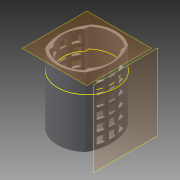
# Autodesk Inventor part: Lattice
Saved by Autodesk Inventor 2013 (Build 170138000, 138)
## iProperties
Created: 2014-07-04
Part Number: Lattice
Material: Genérico
Document SubType Name: Chapa
Designer: Administrador
Density: 1 g/cm^3
Sheet Metal Rule: Por defecto_mm
Author: Administrador
Autodesk Inventor part; units mm, degrees
ref_plane "XZ Plane" through (0, 0, 0) normal (0, 1, 0) x (-1, 0, 0)
ref_plane "XY Plane" through (0, 0, 0) normal (0, 0, 1) x (1, 0, 0)
sketch "Boceto1" plane through (0, 0, 0) normal (0, 0, 1) x (1, 0, 0)
  circle A0 centre (0, 0) radius 20.1
  circle A1 centre (0, 0) radius 18.1
  line L0 (-13, 22.4256) -> (13, 22.4256)
  line L1 (13, 22.4256) -> (13, -22.4256)
  line L2 (13, -22.4256) -> (-13, -22.4256)
  line L3 (-13, -22.4256) -> (-13, 22.4256)
  line L4 (-13, 22.4256) -> (13, -22.4256) construction
  line L5 (13, 22.4256) -> (-13, -22.4256) construction
  circle A2 centre (0, 0) radius 22.1
  dimension "d0" = 40.2
  dimension "d1" = 36.2
  dimension "d2" = 26
  dimension "d3" = 44.2
  constraints: 12 end point, 3 centre point, 2 midpoint, 2 parallel, 1 horizontal, 1 perpendicular
  measures "d0" diameter of A0
  measures "d1" diameter of A1
  measures "d2" distance of L1.end L2.end
  measures "d3" diameter of A2
extrude "Extrusión1" add sketch "Boceto1" along normal blind 10 contours A0 L1 A1 | A0 L1 A2 | L1 A1 L3 A0 | A0 L3 A2 L1 | L1 A2 L3 A0 | A0 L3 A1 L1 | L3 A1 A0 | A0 L3 A2
sketch "Boceto2" plane through (0, 0, 10) normal (0, 0, 1) x (1, 0, 0)
  line L0 (-13.4694, 30.192) -> (13.3129, 30.192)
  line L1 (13.3129, 30.192) -> (13.3129, -30.5468)
  line L2 (13.3129, -30.5468) -> (-13.4694, -30.5468)
  line L3 (-13.4694, -30.5468) -> (-13.4694, 30.192)
  line L4 (-13.4694, 30.192) -> (13.3129, -30.5468) construction
  line L5 (13.3129, 30.192) -> (-13.4694, -30.5468) construction
  circle A0 centre (0, 0) radius 22.0966
  line L6 (-13, 18.1) -> (-15.3267, 9.6283)
  line L7 (13, 18.1) -> (15.412, 9.491)
  line L8 (13, -18.1) -> (15.608, -9.1652)
  line L9 (-13, -18.1) -> (-15.3267, -9.1652)
  arc A1 (13.3129, 15.0591) -> (-13.4694, 14.9193) centre (0, 0) ccw
  arc A2 (14.1027, -14.3221) -> (14.0417, 14.382) centre (0, 0) ccw
  arc A3 (-14.0136, 14.4093) -> (-13.9434, -14.4773) centre (0, 0) ccw
  arc A4 (-13.4694, -14.9193) -> (13.3129, -15.0591) centre (0, 0) ccw
  point P0 (-0.0782, -0.1774)
  dimension "d32" = 26.7823
  constraints: 20 end point, 8 point on circle, 8 point on line, 5 centre point, 2 midpoint, 2 parallel, 1 horizontal, 1 perpendicular
  measures "d32" distance of L1.end L2.end
extrude "Extrusión2" cut sketch "Boceto2" against normal through all contours A1 L1 A4 L3
sketch "Boceto3" plane through (0, 0, 10) normal (0, 0, 1) x (1, 0, 0)
  circle A0 centre (0, 0) radius 22.1 projected
  line L0 (13.3129, -12.2628) -> (13.3129, -15.0591) projected
  arc A1 (-13.4694, -14.9193) -> (13.3129, -15.0591) centre (0, 0) ccw projected
  line L1 (-13.4694, -14.9193) -> (-13.4694, -12.0907) projected
  arc A2 (-13.4694, 12.0907) -> (-13.4694, -12.0907) centre (0, 0) ccw projected
  line L2 (-13.4694, 12.0907) -> (-13.4694, 14.9193) projected
  arc A3 (13.3129, 15.0591) -> (-13.4694, 14.9193) centre (0, 0) ccw projected
  line L3 (13.3129, 15.0591) -> (13.3129, 12.2628) projected
  arc A4 (13.3129, -12.2628) -> (13.3129, 12.2628) centre (0, 0) ccw projected
ref_plane "Plano de trabajo1" through (0, 0, 24.5) normal (0, 0, 1) x (1, 0, 0)
sketch "Boceto5" plane through (0, 0, 24.5) normal (0, 0, 1) x (1, 0, 0)
  circle A0 centre (0, 0) radius 22.1 projected
  arc A1 (13.3129, 15.0591) -> (-13.4694, 14.9193) centre (0, 0) ccw projected
  line L0 (-13.4694, 12.0907) -> (-13.4694, 14.9193) projected
  arc A2 (-13.4694, 12.0907) -> (-13.4694, -12.0907) centre (0, 0) ccw projected
  line L1 (-13.4694, -14.9193) -> (-13.4694, -12.0907) projected
  arc A3 (-13.4694, -14.9193) -> (13.3129, -15.0591) centre (0, 0) ccw projected
  line L2 (13.3129, -12.2628) -> (13.3129, -15.0591) projected
  arc A4 (13.3129, -12.2628) -> (13.3129, 12.2628) centre (0, 0) ccw projected
  line L3 (13.3129, 15.0591) -> (13.3129, 12.2628) projected
  line L4 (-0.172, 27.8672) -> (-0.172, -32.3033)
  arc A5 (13.2871, -19.3756) -> (13.9152, 16.5315) centre (0.9992, -1.2016) ccw
  arc A6 (-12.5238, 19.0209) -> (-13.9692, -18.7386) centre (12.6013, -0.8483) ccw
  arc A7 (-12.5238, 19.0209) -> (-13.9692, -18.7386) centre (-2.0748, -0.2865) ccw
  arc A8 (13.6252, -18.7386) -> (12.1797, 19.0209) centre (-12.9453, -0.8483) ccw
  arc A9 (13.6252, -18.7386) -> (12.1797, 19.0209) centre (1.7308, -0.2865) ccw
  constraints: 10 point on circle, 5 centre point, 4 symmetric about line, 2 end point, 2 other
extrude "Extrusión4" cut sketch "Boceto5" against normal through all contours A0 A8 A5 | A0 A5 A9 A8 | A5 A8 A0 | A0 A8 A9 A5 | A6 A7 A0 | A0 A6
sketch "Boceto6" plane through (0, 0, 24.5) normal (0, 0, 1) x (1, 0, 0)
  line L0 (13.3129, -12.2628) -> (13.3129, -15.0591) projected
  arc A0 (-13.4694, -14.9193) -> (13.3129, -15.0591) centre (0, 0) ccw projected
  line L1 (-13.4694, -14.9193) -> (-13.4694, -12.0907) projected
  arc A1 (-13.4694, 12.0907) -> (-13.4694, -12.0907) centre (0, 0) ccw projected
  line L2 (-13.4694, 12.0907) -> (-13.4694, 14.9193) projected
  arc A2 (13.3129, 15.0591) -> (-13.4694, 14.9193) centre (0, 0) ccw projected
  line L3 (13.3129, 15.0591) -> (13.3129, 12.2628) projected
  arc A3 (13.3129, -12.2628) -> (13.3129, 12.2628) centre (0, 0) ccw projected
  arc A4 (15.3099, -15.9379) -> (13.0991, 17.7996) centre (-12.9453, -0.8483) ccw projected
  arc A5 (13.0991, 17.7996) -> (-13.844, 17.2266) centre (0, 0) ccw projected
  arc A6 (-13.844, 17.2266) -> (-16.028, -15.2156) centre (12.6013, -0.8483) ccw projected
  arc A7 (-16.028, -15.2156) -> (15.3099, -15.9379) centre (0, 0) ccw projected
extrude "Extrusión5" add sketch "Boceto6" against normal blind 52
ref_plane "Plano de trabajo2" through (29, 0, 0) normal (1, 0, 0) x (0, 1, 0)
sketch "Boceto7" plane through (29, 0, 0) normal (1, 0, 0) x (0, 1, 0)
  line L0 (17.7996, 24.5) -> (-15.9379, 24.5) projected
  line L1 (-15.2156, 24.5) -> (-22.1, 24.5) projected
  line L2 (-22.1, -27.5) -> (-22.1, 24.5) projected
  line L3 (22.1, -27.5) -> (22.1, 24.5) projected
  line L4 (22.1, 24.5) -> (17.2266, 24.5) projected
  line L5 (-15.9379, -27.5) -> (17.7996, -27.5) projected
  line L6 (17.2266, -27.5) -> (22.1, -27.5) projected
  line L7 (-22.1, -27.5) -> (-15.2156, -27.5) projected
  line L8 (-15.9379, -27.5) -> (-15.9379, 24.5) projected
  line L9 (17.7996, 24.5) -> (17.7996, -27.5) projected
  line L10 (-12.0907, 24.5) -> (-12.0907, -27.5) projected
  line L11 (12.0907, -27.5) -> (12.0907, 24.5) projected
  line L12 (-10.3756, 20.6878) -> (-5.3756, 20.6878)
  line L13 (-5.3756, 20.6878) -> (-5.3756, 15.6878)
  line L14 (-5.3756, 15.6878) -> (-10.3756, 15.6878)
  line L15 (-10.3756, 15.6878) -> (-10.3756, 20.6878)
  line L16 (-2.3756, 20.6878) -> (2.6244, 20.6878)
  line L17 (2.6244, 20.6878) -> (2.6244, 15.6878)
  line L18 (2.6244, 15.6878) -> (-2.3756, 15.6878)
  line L19 (-2.3756, 15.6878) -> (-2.3756, 20.6878)
  line L20 (5.6244, 20.6878) -> (10.6244, 20.6878)
  line L21 (10.6244, 20.6878) -> (10.6244, 15.6878)
  line L22 (10.6244, 15.6878) -> (5.6244, 15.6878)
  line L23 (5.6244, 15.6878) -> (5.6244, 20.6878)
  line L24 (-10.3756, 12.6878) -> (-5.3756, 12.6878)
  line L25 (-5.3756, 12.6878) -> (-5.3756, 7.6878)
  line L26 (-5.3756, 7.6878) -> (-10.3756, 7.6878)
  line L27 (-10.3756, 7.6878) -> (-10.3756, 12.6878)
  line L28 (-2.3756, 12.6878) -> (2.6244, 12.6878)
  line L29 (2.6244, 12.6878) -> (2.6244, 7.6878)
  line L30 (2.6244, 7.6878) -> (-2.3756, 7.6878)
  line L31 (-2.3756, 7.6878) -> (-2.3756, 12.6878)
  line L32 (5.6244, 12.6878) -> (10.6244, 12.6878)
  line L33 (10.6244, 12.6878) -> (10.6244, 7.6878)
  line L34 (10.6244, 7.6878) -> (5.6244, 7.6878)
  line L35 (5.6244, 7.6878) -> (5.6244, 12.6878)
  line L36 (-10.3756, 4.6878) -> (-5.3756, 4.6878)
  line L37 (-5.3756, 4.6878) -> (-5.3756, -0.3122)
  line L38 (-5.3756, -0.3122) -> (-10.3756, -0.3122)
  line L39 (-10.3756, -0.3122) -> (-10.3756, 4.6878)
  line L40 (-2.3756, 4.6878) -> (2.6244, 4.6878)
  line L41 (2.6244, 4.6878) -> (2.6244, -0.3122)
  line L42 (2.6244, -0.3122) -> (-2.3756, -0.3122)
  line L43 (-2.3756, -0.3122) -> (-2.3756, 4.6878)
  line L44 (5.6244, 4.6878) -> (10.6244, 4.6878)
  line L45 (10.6244, 4.6878) -> (10.6244, -0.3122)
  line L46 (10.6244, -0.3122) -> (5.6244, -0.3122)
  line L47 (5.6244, -0.3122) -> (5.6244, 4.6878)
  line L48 (-10.3756, -3.3122) -> (-5.3756, -3.3122)
  line L49 (-5.3756, -3.3122) -> (-5.3756, -8.3122)
  line L50 (-5.3756, -8.3122) -> (-10.3756, -8.3122)
  line L51 (-10.3756, -8.3122) -> (-10.3756, -3.3122)
  line L52 (-2.3756, -3.3122) -> (2.6244, -3.3122)
  line L53 (2.6244, -3.3122) -> (2.6244, -8.3122)
  line L54 (2.6244, -8.3122) -> (-2.3756, -8.3122)
  line L55 (-2.3756, -8.3122) -> (-2.3756, -3.3122)
  line L56 (5.6244, -3.3122) -> (10.6244, -3.3122)
  line L57 (10.6244, -3.3122) -> (10.6244, -8.3122)
  line L58 (10.6244, -8.3122) -> (5.6244, -8.3122)
  line L59 (5.6244, -8.3122) -> (5.6244, -3.3122)
  line L60 (-10.3756, -11.3122) -> (-5.3756, -11.3122)
  line L61 (-5.3756, -11.3122) -> (-5.3756, -16.3122)
  line L62 (-5.3756, -16.3122) -> (-10.3756, -16.3122)
  line L63 (-10.3756, -16.3122) -> (-10.3756, -11.3122)
  line L64 (-2.3756, -11.3122) -> (2.6244, -11.3122)
  line L65 (2.6244, -11.3122) -> (2.6244, -16.3122)
  line L66 (2.6244, -16.3122) -> (-2.3756, -16.3122)
  line L67 (-2.3756, -16.3122) -> (-2.3756, -11.3122)
  line L68 (5.6244, -11.3122) -> (10.6244, -11.3122)
  line L69 (10.6244, -11.3122) -> (10.6244, -16.3122)
  line L70 (10.6244, -16.3122) -> (5.6244, -16.3122)
  line L71 (5.6244, -16.3122) -> (5.6244, -11.3122)
  line L72 (-10.3756, -19.3122) -> (-5.3756, -19.3122)
  line L73 (-5.3756, -19.3122) -> (-5.3756, -24.3122)
  line L74 (-5.3756, -24.3122) -> (-10.3756, -24.3122)
  line L75 (-10.3756, -24.3122) -> (-10.3756, -19.3122)
  line L76 (-2.3756, -19.3122) -> (2.6244, -19.3122)
  line L77 (2.6244, -19.3122) -> (2.6244, -24.3122)
  line L78 (2.6244, -24.3122) -> (-2.3756, -24.3122)
  line L79 (-2.3756, -24.3122) -> (-2.3756, -19.3122)
  line L80 (5.6244, -19.3122) -> (10.6244, -19.3122)
  line L81 (10.6244, -19.3122) -> (10.6244, -24.3122)
  line L82 (10.6244, -24.3122) -> (5.6244, -24.3122)
  line L83 (5.6244, -24.3122) -> (5.6244, -19.3122)
  point P0 (0, 0)
  dimension "d20" = 5
  dimension "d21" = 5
  dimension "d24" = 8
  dimension "d27" = 8
  constraints: 144 end point, 2 horizontal, 2 parallel, 1 perpendicular, 1 vertical, 136 other
  measures "d20" distance of L13.end L14.end
  measures "d21" distance of L12.end L13.end
  measures "d24" distance of L12.start L16.start
  measures "d27" distance of L12.start L24.start
extrude "Extrusión6" cut sketch "Boceto7" against normal through all contours L12 L13 L14 L15 | L16 L17 L18 L19 | L20 L21 L22 L23 | L24 L25 L26 L27 | L28 L29 L30 L31 | L32 L33 L34 L35 | L36 L37 L38 L39 | L40 L41 L42 L43 | L44 L45 L46 L47 | L48 L49 L50 L51 | L52 L53 L54 L55 | L56 L57 L58 L59 | L60 L61 L62 L63 | L64 L65 L66 L67 | L68 L69 L70 L71 | L72 L73 L74 L75 | L76 L77 L78 L79 | L80 L81 L82 L83
equation "\"Radio_pliegue\" = Grosor"
equation "\"Anchura_desahogo_plegado\" = Grosor"
equation "\"Profundidad_desahogo_plegado\" = 0.5 * Grosor"
equation "\"Tamaño_destalonado\" = 4 * Grosor"
equation "\"Remanente_mínimo\" = 2 * Grosor"
equation "\"Radiodetransición\" = Radio_pliegue"
equation "\"Tamaño_de_radio_de_Jacobi\" = Radio_pliegue"
equation "\"TamañoSeparación\" = Grosor"
equation "\"Grosor\" = 0.5"
